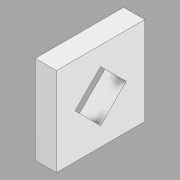
# Autodesk Inventor part: y_axis_mount
Saved by Autodesk Inventor 2020 (Build 240168000, 168)
## iProperties
Created: 2021-04-02
Part Number: y_axis_mount
Material: ABS Plastic
Document SubType Name: Modeling
Designer: griss
Density: 1.06 g/cm^3
Appearance: Smooth - White
Author: griss
Autodesk Inventor part; units mm, degrees
ref_plane "YZ Plane" through (0, 0, 0) normal (1, 0, 0) x (0, 1, 0)
ref_plane "XZ Plane" through (0, 0, 0) normal (0, 1, 0) x (-1, 0, 0)
ref_plane "XY Plane" through (0, 0, 0) normal (0, 0, 1) x (1, 0, 0)
sketch "Sketch1" plane through (0, 0, 0) normal (1, 0, 0) x (0, 1, 0)
  line L0 (0, 17.9605) -> (17.9605, 0) construction
  line L1 (17.9605, 0) -> (0, -17.9605) construction
  line L2 (0, -17.9605) -> (-17.9605, 0) construction
  line L3 (-17.9605, 0) -> (0, 17.9605) construction
  line L4 (0, 17.9605) -> (0, -17.9605) construction
  line L5 (17.9605, 0) -> (-17.9605, 0) construction
  line L6 (0, 18.3816) -> (-18.3816, 0)
  line L7 (0, 18.3816) -> (18.3816, 0)
  line L8 (18.3816, 0) -> (0, -18.3816)
  line L9 (-18.3816, 0) -> (0, -18.3816)
  line L10 (0, 25.5658) -> (-25.5658, 0)
  line L11 (-25.5658, 0) -> (0, -25.5658)
  line L12 (0, -25.5658) -> (25.5658, 0)
  line L13 (25.5658, 0) -> (0, 25.5658)
  line L14 (-44.45, 0) -> (44.45, 0) projected
  line L15 (0, -44.45) -> (0, 44.45) projected
  line L16 (31.75, 31.75) -> (-31.75, 31.75)
  line L17 (-31.75, 31.75) -> (-31.75, -31.75)
  line L18 (-31.75, -31.75) -> (31.75, -31.75)
  line L19 (31.75, -31.75) -> (31.75, 31.75)
  line L20 (31.75, 31.75) -> (-31.75, -31.75) construction
  line L21 (-31.75, 31.75) -> (31.75, -31.75) construction
  point P0 (0, 0)
  point P1 (0, 0)
  point P2 (0, 0)
  point P3 (0, 0)
  point P4 (29.7157, 21.8287)
  point P5 (0, 0)
  dimension "d0" = 25.4
  dimension "d1" = 25.4
  dimension "d3" = 5.08
  dimension "d4" = 5.08
  dimension "d7" = 63.5
  dimension "d8" = 63.5
  constraints: 40 end point, 11 perpendicular, 6 midpoint, 4 parallel, 3 coincident, 2 horizontal alignment, 2 point on line, 1 horizontal, 4 other
  measures "d0" distance of L1.end L2.end
  measures "d1" distance of L0.end L1.end
  measures "d3" distance between parallel lines of L10 L6
  measures "d4" distance between parallel lines of L9 L11
  measures "d7" distance of L18.end L17.end
  measures "d8" distance of L18.end L16.start
extrude "Extrusion1" add sketch "Sketch1" along normal mid plane 15.24 contours L15 L13 L14 L7 | L6 L14 L10 L15 | L9 L15 L11 L14 | L14 L12 L15 L8 | L15 L16 L19 L14 L13 | L10 L14 L17 L16 L15 | L11 L15 L18 L17 L14 | L14 L19 L18 L15 L12
equation "\"d4\" = d3"
equation "\"d8\" = d7"
body "Solid1"
